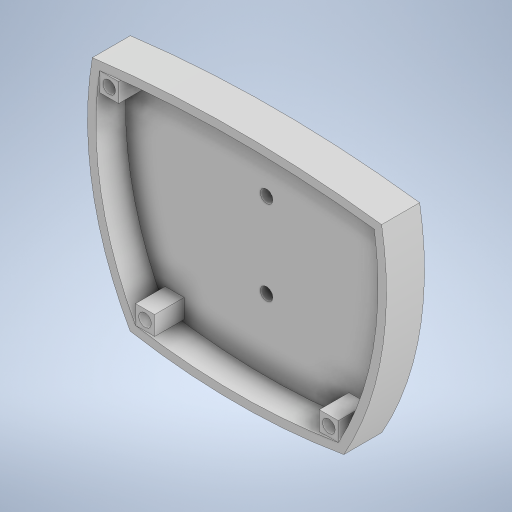
# Autodesk Inventor part: ProjEnAble_Microbit_Cover
Saved by Autodesk Inventor 2023 (Build 270158000, 158)
## iProperties
Created: 2022-11-30
Part Number: ProjEnAble_Microbit_Cover
Material: Generic
Document SubType Name: Modeling
Designer: jeron
Density: 1 g/cm^3
Appearance: Default
Author: jeron
Autodesk Inventor part; units mm, degrees
ref_plane "YZ Plane" through (0, 0, 0) normal (1, 0, 0) x (0, 1, 0)
ref_plane "XZ Plane" through (0, 0, 0) normal (0, 1, 0) x (-1, 0, 0)
ref_plane "XY Plane" through (0, 0, 0) normal (0, 0, 1) x (1, 0, 0)
sketch "Sketch1" plane through (0, 0, 0) normal (0, 0, 1) x (1, 0, 0)
  line L0 (0, 0) -> (0, 23)
  line L1 (0, 0) -> (0, -25)
  line L2 (0, 0) -> (-32.5, 0)
  line L3 (0, 0) -> (32.5, 0)
  line L4 (0, 23) -> (0, 25)
  line L5 (0, -25) -> (0, -27)
  arc A0 (32.5, 23) -> (-32.5, 23) centre (0, -240.0625) ccw
  arc A1 (-24, -25) -> (24, -25) centre (0, 118) ccw
  arc A2 (-34.2324, 24.7969) -> (-25.28, -26.8099) centre (42.3382, 11.5) ccw
  arc A3 (34.2324, 24.7969) -> (-34.2324, 24.7969) centre (0, -240.0625) ccw
  arc A4 (25.28, -26.8099) -> (34.2324, 24.7969) centre (-42.3382, 11.5) ccw
  arc A5 (-25.28, -26.8099) -> (25.28, -26.8099) centre (0, 118) ccw
  line L6 (-27.5, 23) -> (-27.5, 23.5696)
  line L7 (-27.2519, -23.0989) -> (-25.5309, -23.099)
  arc A6 (-32.5, 23) -> (-26.1342, -20.8192) centre (42.3382, 11.5) ccw
  arc A7 (26.1342, -20.8192) -> (32.5, 23) centre (-42.3382, 11.5) ccw
  arc A8 (24, -25) -> (26.1342, -20.8192) centre (-42.3382, 11.5) ccw
  arc A9 (-26.1342, -20.8192) -> (-24, -25) centre (42.3382, 11.5) ccw
  line L8 (-24, -25) -> (-19.5, -25)
  line L9 (-19.5, -25) -> (-19.5, -20.5)
  line L10 (-19.5, -20.5) -> (-24, -20.5)
  line L11 (-24, -20.5) -> (-24, -25)
  line L12 (24, -25) -> (24, -20.5)
  line L13 (24, -20.5) -> (19.5, -20.5)
  line L14 (19.5, -20.5) -> (19.5, -25)
  line L15 (19.5, -25) -> (24, -25)
  circle A10 centre (21.75, -22.75) radius 1.5
  circle A11 centre (-21.75, -22.75) radius 1.5
  line L16 (0, 0) -> (0, 10)
  line L17 (0, 0) -> (0, -10)
  circle A12 centre (0, -10) radius 1.5
  circle A13 centre (0, 10) radius 1.5
  line L18 (-32.5, 23) -> (-28, 23)
  line L19 (-28, 23) -> (-28, 18.5)
  line L20 (-28, 18.5) -> (-32.5, 18.5)
  line L21 (-32.5, 18.5) -> (-32.5, 23)
  circle A14 centre (-30.25, 20.75) radius 1.5
  point P0 (24, -25)
  point P1 (24, -25)
  point P2 (-24, -25)
  point P3 (-24, -25)
  dimension "d0" = 23
  dimension "d1" = 25
  dimension "d4" = 65
  dimension "d6" = 48
  dimension "d7" = 32.5
  dimension "d8" = 32.5
  dimension "d9" = 2
  dimension "d10" = 2
  dimension "d15" = 5
  dimension "d19" = 1.721
  dimension "d33" = 4.5
  dimension "d34" = 4.5
  dimension "d35" = 4.5
  dimension "d36" = 4.5
  dimension "d37" = 4.5
  dimension "d38" = 4.5
  dimension "d43" = 3
  dimension "d44" = 3
  dimension "d51" = 10
  dimension "d52" = 10
  dimension "d53" = 3
  dimension "d54" = 3
  constraints: 44 end point, 28 point on circle, 15 centre point, 6 vertical, 4 horizontal, 4 perpendicular, 2 coincident, 2 concentric, 2 point on line, 1 symmetric about line
  measures "d0" distance of L0.start L0.end
  measures "d1" distance of L0.start L1.end
  measures "d4" distance of L18.start A0.start
  measures "d6" distance of L12.start A1.start
  measures "d7" distance of L0.start L2.end
  measures "d8" distance of L0.start L3.end
  measures "d9" distance of L0.end L4.end
  measures "d10" distance of L1.end L5.end
  measures "d15" distance of L18.start L6.start
  measures "d19" distance of L7.start L7.end
  measures "d33" distance of L8.start L8.end
  measures "d34" distance of L8.end L9.end
  measures "d35" distance of L9.end L10.end
  measures "d36" distance of L12.start L12.end
  measures "d37" distance of L12.end L13.end
  measures "d38" distance of L13.end L14.end
  measures "d43" diameter of A10
  measures "d44" diameter of A11
  measures "d51" distance of L0.start L16.end
  measures "d52" distance of L0.start L17.end
  measures "d53" diameter of A12
  measures "d54" diameter of A13
extrude "Extrusion5" add sketch "Sketch1" against normal blind 2 contours L18 L19 L20 L21 | L2 A6 A0 L4 L0 A13 | L15 L14 L13 L12 | L3 A7 A8 A1 L5 L1 A12 | L11 L10 L9 L8 | L1 A12 L5 A1 A9 A6 L2 | L0 A13 L4 A0 A7 L3 | A13 L0 | L0 A13 | A12 L1 | L1 A12 | A3 A4 A5 A2 | A10 | A11 | A14
extrude "Extrusion6" add sketch "Sketch1" along normal blind 7
extrude "Extrusion7" cut sketch "Sketch1" against normal blind 2 contours A10 | A11
extrude "Extrusion8" cut sketch "Sketch1" against normal through all contours A13 L0 | L0 A13 | A12 L1 | L1 A12
extrude "Extrusion9" cut sketch "Sketch1" against normal through all contours A14
body "Solid2"
